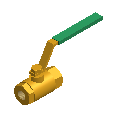
# Autodesk Inventor part: Parker Female-Female Pipe Ends XV500P XV500P-12
Saved by Autodesk Inventor 2020 (Build 240152000, 152)
## iProperties
_DisabledCommands: 0
Created: 2009-02-04
Part Number: Parker Female-Female Pipe Ends XV500P XV500P-12
Material: Brass, Soft Yellow
Description: Female-Female Pipe Ends
Document SubType Name: Modeling
Standard: Parker
Designer: Demir Ali
Manufacturer: Parker
Language: en-US
Size Designation: XV500P-12
Categories: <MemberInstance><Categories><Category DisplayName="Tube &amp; Pipe" InternalName="4347fa0f-2144-441d-94cd-e3e15c92b736" Mnemonic="TUBEANDPIPE"><CategoryParameter DisplayName="InLineGroups" InternalName="d60be647-bc43-4c18-a13f-9fe4115f8e64" Mnemonic="INLINEGROUPS"/><CategoryParameter DisplayName="Number of Connections" InternalName="04e9c83a-9e20-4a98-a7e1-e8abe87a2846" Mnemonic="NUM_CONNECTIONS"/><CategoryParameter DisplayName="Angles" InternalName="0e0e4fa4-3bd3-4656-a22e-4e07c8c476f8" Mnemonic="ANGLES"><CategoryParameter DisplayName="Angle" InternalName="9188ad83-1b16-48b4-8b0a-76ce729dafa7" Mnemonic="ANGLE"/></CategoryParameter><CategoryParameter DisplayName="NameOfComponent" InternalName="9c74ad13-48a1-45fe-b0f7-5447561f444a" Mnemonic="NAMEOFCOMPONENT"/><CategoryParameter DisplayName="SKey" InternalName="3da84699-049a-4bc2-a65a-6696b77c242f" Mnemonic="SKEY"/><CategoryParameter DisplayName="ITEM-CODE" InternalName="99cc3b15-24d9-4d38-aac7-792cfbc57acf" Mnemonic="ITEMCODE"/><CategoryParameter DisplayName="ISOGEN Description" InternalName="7aa3ba45-b821-4467-8584-f9e6f15f2a7d" Mnemonic="ISOGENDESC"/><Category DisplayName="Fittings" InternalName="ed6b26c4-72b8-4f31-9b63-f85ae8f932e4" Mnemonic="FITTINGS"><CategoryParameter DisplayName="Connections" InternalName="dbd721e8-e885-4eea-9011-b5acfd9f61de" Mnemonic="FIT_CONNECTIONS"><CategoryParameter DisplayName="NominalSize" InternalName="3f94edc7-e459-48db-8f02-8eebf8cffccd" Mnemonic="NS"/><CategoryParameter DisplayName="FlipDirection" InternalName="d55dedc0-f14a-4283-86b4-a4eeb253c8aa" Mnemonic="FLIPDIRECTION"/><CategoryParameter DisplayName="DisplayName" InternalName="50f521dd-e050-43f7-9895-6b30ea7ed42e" Mnemonic="DISPLAYNAME"/><CategoryParameter DisplayName="Female" InternalName="b366bcb5-a500-4bad-84bb-22f956216d69" Mnemonic="FEMALE"/><CategoryParameter DisplayName="EndTreatment" InternalName="d7f11516-3374-45ca-b1c7-4b2d63244ae2" Mnemonic="ENDTREATMENT"/><CategoryParameter DisplayName="Fixed" InternalName="9142902a-6a8a-446d-9eb8-4b7ce7d245ef" Mnemonic="FIXED"/><CategoryParameter DisplayName="MaxEngagement" InternalName="34fdf028-8797-436e-ba07-ca3dee15bd9b" Mnemonic="MAXENGAGEMENT"/><CategoryParameter DisplayName="MinEngagement [% of MaxEngagement]" InternalName="7ec1bde5-73f0-45b1-98d8-365a6c67f8ad" Mnemonic="MINENGAGEMENT"/><CategoryParameter DisplayName="ScheduleNumber" InternalName="d6161c62-eb59-4495-a086-874847c10866" Mnemonic="SN"/><CategoryParameter DisplayName="Max Mating Pipe Size" InternalName="e73ef66b-c04b-45ac-9b32-f712653e25ee" Mnemonic="MXMPS"/><CategoryParameter DisplayName="Min Mating Pipe Size" InternalName="11f51b32-3e37-4310-abf7-f1318a1fd129" Mnemonic="MNMPS"/><CategoryParameter DisplayName="Cut Mating Pipe" InternalName="53a63a6e-53d8-4ca9-8880-037731d1cceb" Mnemonic="CMP"/><CategoryParameter DisplayName="Gender Neutral" InternalName="628bd5f1-acad-44e2-9d91-af996ab74fc2" Mnemonic="NEUTRAL"/></CategoryParameter><CategoryParameter DisplayName="Connections" InternalName="dbd721e8-e885-4eea-9011-b5acfd9f61de" Mnemonic="FIT_CONNECTIONS"><CategoryParameter DisplayName="NominalSize" InternalName="3f94edc7-e459-48db-8f02-8eebf8cffccd" Mnemonic="NS"/><CategoryParameter DisplayName="FlipDirection" InternalName="d55dedc0-f14a-4283-86b4-a4eeb253c8aa" Mnemonic="FLIPDIRECTION"/><CategoryParameter DisplayName="DisplayName" InternalName="50f521dd-e050-43f7-9895-6b30ea7ed42e" Mnemonic="DISPLAYNAME"/><CategoryParameter DisplayName="Female" InternalName="b366bcb5-a500-4bad-84bb-22f956216d69" Mnemonic="FEMALE"/><CategoryParameter DisplayName="EndTreatment" InternalName="d7f11516-3374-45ca-b1c7-4b2d63244ae2" Mnemonic="ENDTREATMENT"/><CategoryParameter DisplayName="Fixed" InternalName="9142902a-6a8a-446d-9eb8-4b7ce7d245ef" Mnemonic="FIXED"/><CategoryParameter DisplayName="MaxEngagement" InternalName="34fdf028-8797-436e-ba07-ca3dee15bd9b" Mnemonic="MAXENGAGEMENT"/><CategoryParameter DisplayName="MinEngagement [% of MaxEngagement]" InternalName="7ec1bde5-73f0-45b1-98d8-365a6c67f8ad" Mnemonic="MINENGAGEMENT"/><CategoryParameter DisplayName="ScheduleNumber" InternalName="d6161c62-eb59-4495-a086-874847c10866" Mnemonic="SN"/><CategoryParameter DisplayName="Max Mating Pipe Size" InternalName="e73ef66b-c04b-45ac-9b32-f712653e25ee" Mnemonic="MXMPS"/><CategoryParameter DisplayName="Min Mating Pipe Size" InternalName="11f51b32-3e37-4310-abf7-f1318a1fd129" Mnemonic="MNMPS"/><CategoryParameter DisplayName="Cut Mating Pipe" InternalName="53a63a6e-53d8-4ca9-8880-037731d1cceb" Mnemonic="CMP"/><CategoryParameter DisplayName="Gender Neutral" InternalName="628bd5f1-acad-44e2-9d91-af996ab74fc2" Mnemonic="NEUTRAL"/></CategoryParameter><Category DisplayName="Valves" InternalName="b54f24b4-8c71-4f76-b075-760a31c67e8e" Mnemonic="Valve"/></Category></Category><Category DisplayName="DataType" InternalName="23b78d0f-2648-40c6-8793-ca6db495c9e8" Mnemonic="DATATYPE"><CategoryParameter DisplayName="DisplayName" InternalName="05415f3d-3907-474b-a020-eb9d644f4cf3" Mnemonic="DISPLAYNAME"/><CategoryParameter DisplayName="InternalName" InternalName="cf1d0246-76d9-4b4a-8305-fa0409afb5c1" Mnemonic="INTERNALNAME"/><CategoryParameter DisplayName="Folder Name" InternalName="3f06958e-8713-4116-9be7-ed6184ecc97b" Mnemonic="FOLDERNAME"/><CategoryParameter DisplayName="Family Version" InternalName="914462f6-6e19-4b14-ba84-155b9680b1d0" Mnemonic="FAMILYREVISION"/><CategoryParameter DisplayName="ClipFormat" InternalName="bc51e27b-3422-4e78-93ef-cec197ddf230" Mnemonic="CLIPFORMAT"/><CategoryParameter DisplayName="IsMetric" InternalName="e2385c5b-1ea4-4823-96a8-8de651266ec3" Mnemonic="ISMETRIC"/><CategoryParameter DisplayName="Description" InternalName="13903e3d-64b1-4950-80da-f627842ea37f" Mnemonic="DESCRIPTION"/><CategoryParameter DisplayName="StdsOrg" InternalName="8f5914e1-4693-403f-8ab5-d37768198c9d" Mnemonic="STDSORG"/><CategoryParameter DisplayName="Standard" InternalName="0c0a119c-1e12-4c84-803f-101930972f5e" Mnemonic="STANDARD"/><CategoryParameter DisplayName="Manufacturer" InternalName="cd6c7a72-a28a-4e50-99a9-2c7f4e13e5ad" Mnemonic="MANUFACTURER"/><CategoryParameter DisplayName="Member Revision" InternalName="a65d44b9-392f-4f4f-857b-e4b3d54996fe" Mnemonic="MEMBERREVISION"/><CategoryParameter DisplayName="Standard Revision" InternalName="91d5a463-65c2-4fde-b823-3b7fea5e8e17" Mnemonic="STANDARDREVISION"/><CategoryParameter DisplayName="Revision Guid" InternalName="45a75005-10b1-4dfc-8d6d-dfe629f0b93c" Mnemonic="REVISIONGUID"/><CategoryParameter DisplayName="Designation" InternalName="2675968c-4ce5-49e0-a4f5-552d29089031" Mnemonic="DESIGNATION"/><CategoryParameter DisplayName="FileName" InternalName="8b46a4cc-9585-4fed-90c3-899f57e09a73" Mnemonic="FILENAME"/><CategoryParameter DisplayName="Default Row" InternalName="2af9ec52-faaa-4026-b378-f9fa4afca842" Mnemonic="DEFAULTROW"/><Category DisplayName="Part" InternalName="c0e0b642-3bcb-4cc8-9e80-f96d35c4afa4" Mnemonic="PART"><CategoryParameter DisplayName="Material" InternalName="818a152a-d3c3-49ca-80ee-df7d91421b8e" Mnemonic="MATERIAL"/><CategoryParameter DisplayName="Material Key" InternalName="5c9a8adb-dd2b-4535-b97f-0a94a95fe41f" Mnemonic="MATERIALKEY"/><CategoryParameter DisplayName="Part Number" InternalName="016b6077-bfbe-49bd-92c9-d8d59c39c941" Mnemonic="PARTNUMBER"/><CategoryParameter DisplayName="Stock Number" InternalName="4dba7c1c-e26c-444e-836c-b08b433409a8" Mnemonic="STOCKNUMBER"/></Category></Category><Category DisplayName="LegacyMap" InternalName="dfeab48a-acc2-4514-a11c-1b8dc28c3d5f" Mnemonic="LEGACYMAP"><CategoryParameter DisplayName="CatalogID" InternalName="0da51c36-8fd3-4028-86cc-0c9c9e96136a" Mnemonic="CATALOGID"/><CategoryParameter DisplayName="FamilyID" InternalName="1c0b589c-8bbe-4e1e-80cf-07c0de42ac2a" Mnemonic="FAMILYID"/><CategoryParameter DisplayName="MemberID" InternalName="a368ea03-db8a-4d6e-962b-2aa46306b8f5" Mnemonic="MEMBERID"/></Category></Categories><FamilyTemplate Id="Parker Female-Female Pipe Ends XV500P"><FamilyTemplateParameters><FamilyTemplateParameter ObjectType="kUserParameterObject" ValueType="xs:double" Id="1" ObjectReferenceKey="D"/><FamilyTemplateParameter ObjectType="kUserParameterObject" ValueType="xs:double" Id="2" ObjectReferenceKey="N1"/><FamilyTemplateParameter ObjectType="kUserParameterObject" ValueType="xs:double" Id="3" ObjectReferenceKey="M"/><FamilyTemplateParameter ObjectType="kUserParameterObject" ValueType="xs:double" Id="4" ObjectReferenceKey="H1"/><FamilyTemplateParameter ObjectType="kUserParameterObject" ValueType="xs:double" Id="5" ObjectReferenceKey="L"/><FamilyTemplateParameter ObjectType="kUserParameterObject" ValueType="xs:double" Id="6" ObjectReferenceKey="B_HEX"/><FamilyTemplateParameter ObjectType="kUserParameterObject" ValueType="xs:double" Id="7" ObjectReferenceKey="C_HEX"/><FamilyTemplateParameter ObjectType="kUserParameterObject" ValueType="xs:string" Id="118" ObjectReferenceKey="Parker_No"/><FamilyTemplateParameter ObjectType="kPropertyObject" ValueType="xs:string" Id="100" ObjectReferenceKey="{32853F0F-3444-11d1-9E93-0060B03C1CA6}" SubObjectId="52"/><FamilyTemplateParameter ObjectType="kPropertyObject" ValueType="xs:string" Id="105" ObjectReferenceKey="{32853F0F-3444-11d1-9E93-0060B03C1CA6}" SubObjectId="5"/><FamilyTemplateParameter ObjectType="kPartComponentDefinitionObject" ValueType="xs:string" Id="110" SubObjectId="Material"/><FamilyTemplateParameter ObjectType="kThreadFeatureObject" ValueType="xs:structure" Id="300" ObjectReferenceKey="10020000100000002B880000000000008000000000000000" SubObjectId="ThreadInfo"><FamilyTemplateParameter ObjectType="" ValueType="xs:string" Id="301" SubObjectId="ThreadType"/><FamilyTemplateParameter ObjectType="" ValueType="xs:string" Id="302" SubObjectId="NominalDiameter"/></FamilyTemplateParameter><FamilyTemplateParameter ObjectType="kThreadFeatureObject" ValueType="xs:structure" Id="303" ObjectReferenceKey="100200001000000095880000000000008000000000000000" SubObjectId="ThreadInfo"><FamilyTemplateParameter ObjectType="" ValueType="xs:string" Id="304" SubObjectId="ThreadType"/><FamilyTemplateParameter ObjectType="" ValueType="xs:string" Id="305" SubObjectId="NominalDiameter"/></FamilyTemplateParameter></FamilyTemplateParameters></FamilyTemplate><CategoryParameterMap><ParamToTemplateMap><ParamToTemplate CategoryParameter="//CategoryParameter[@InternalName='d60be647-bc43-4c18-a13f-9fe4115f8e64']" ConstantValue="1"/><ParamToTemplate CategoryParameter="//CategoryParameter[@InternalName='04e9c83a-9e20-4a98-a7e1-e8abe87a2846']" ConstantValue="2"/><ParamToTemplate CategoryParameter="//CategoryParameter[@InternalName='0e0e4fa4-3bd3-4656-a22e-4e07c8c476f8']" ConstantValue=""/><ParamToTemplate CategoryParameter="//CategoryParameter[@InternalName='0e0e4fa4-3bd3-4656-a22e-4e07c8c476f8'][1]/CategoryParameter[@InternalName='9188ad83-1b16-48b4-8b0a-76ce729dafa7']" ConstantValue="3.14159265358979"/><ParamToTemplate CategoryParameter="//CategoryParameter[@InternalName='9c74ad13-48a1-45fe-b0f7-5447561f444a']" ConstantValue="VALVE"/><ParamToTemplate CategoryParameter="//CategoryParameter[@InternalName='3da84699-049a-4bc2-a65a-6696b77c242f']" ConstantValue="VBSC"/><ParamToTemplate CategoryParameter="//CategoryParameter[@InternalName='dbd721e8-e885-4eea-9011-b5acfd9f61de'][1]/CategoryParameter[@InternalName='d55dedc0-f14a-4283-86b4-a4eeb253c8aa']" ConstantValue="false"/><ParamToTemplate CategoryParameter="//CategoryParameter[@InternalName='dbd721e8-e885-4eea-9011-b5acfd9f61de'][1]/CategoryParameter[@InternalName='50f521dd-e050-43f7-9895-6b30ea7ed42e']" ConstantValue="Connection1"/><ParamToTemplate CategoryParameter="//CategoryParameter[@InternalName='dbd721e8-e885-4eea-9011-b5acfd9f61de'][1]/CategoryParameter[@InternalName='b366bcb5-a500-4bad-84bb-22f956216d69']" ConstantValue="true"/><ParamToTemplate CategoryParameter="//CategoryParameter[@InternalName='dbd721e8-e885-4eea-9011-b5acfd9f61de'][1]/CategoryParameter[@InternalName='d7f11516-3374-45ca-b1c7-4b2d63244ae2']" ConstantValue="Threaded"/><ParamToTemplate CategoryParameter="//CategoryParameter[@InternalName='dbd721e8-e885-4eea-9011-b5acfd9f61de'][1]/CategoryParameter[@InternalName='9142902a-6a8a-446d-9eb8-4b7ce7d245ef']" ConstantValue="false"/><ParamToTemplate CategoryParameter="//CategoryParameter[@InternalName='dbd721e8-e885-4eea-9011-b5acfd9f61de'][1]/CategoryParameter[@InternalName='34fdf028-8797-436e-ba07-ca3dee15bd9b']" ConstantValue="0"/><ParamToTemplate CategoryParameter="//CategoryParameter[@InternalName='dbd721e8-e885-4eea-9011-b5acfd9f61de'][1]/CategoryParameter[@InternalName='7ec1bde5-73f0-45b1-98d8-365a6c67f8ad']" ConstantValue="50"/><ParamToTemplate CategoryParameter="//CategoryParameter[@InternalName='dbd721e8-e885-4eea-9011-b5acfd9f61de'][2]/CategoryParameter[@InternalName='d55dedc0-f14a-4283-86b4-a4eeb253c8aa']" ConstantValue="false"/><ParamToTemplate CategoryParameter="//CategoryParameter[@InternalName='dbd721e8-e885-4eea-9011-b5acfd9f61de'][2]/CategoryParameter[@InternalName='50f521dd-e050-43f7-9895-6b30ea7ed42e']" ConstantValue="Connection2"/><ParamToTemplate CategoryParameter="//CategoryParameter[@InternalName='dbd721e8-e885-4eea-9011-b5acfd9f61de'][2]/CategoryParameter[@InternalName='b366bcb5-a500-4bad-84bb-22f956216d69']" ConstantValue="true"/><ParamToTemplate CategoryParameter="//CategoryParameter[@InternalName='dbd721e8-e885-4eea-9011-b5acfd9f61de'][2]/CategoryParameter[@InternalName='d7f11516-3374-45ca-b1c7-4b2d63244ae2']" ConstantValue="Threaded"/><ParamToTemplate CategoryParameter="//CategoryParameter[@InternalName='dbd721e8-e885-4eea-9011-b5acfd9f61de'][2]/CategoryParameter[@InternalName='9142902a-6a8a-446d-9eb8-4b7ce7d245ef']" ConstantValue="false"/><ParamToTemplate CategoryParameter="//CategoryParameter[@InternalName='dbd721e8-e885-4eea-9011-b5acfd9f61de'][2]/CategoryParameter[@InternalName='34fdf028-8797-436e-ba07-ca3dee15bd9b']" ConstantValue="0"/><ParamToTemplate CategoryParameter="//CategoryParameter[@InternalName='dbd721e8-e885-4eea-9011-b5acfd9f61de'][2]/CategoryParameter[@InternalName='7ec1bde5-73f0-45b1-98d8-365a6c67f8ad']" ConstantValue="50"/><ParamToTemplate CategoryParameter="//CategoryParameter[@InternalName='05415f3d-3907-474b-a020-eb9d644f4cf3']" ConstantValue="Parker Female-Female Pipe Ends XV500P"/><ParamToTemplate CategoryParameter="//CategoryParameter[@InternalName='cf1d0246-76d9-4b4a-8305-fa0409afb5c1']" ConstantValue="c0da0a2f-7571-4003-bdb7-f2d41c6df3db"/><ParamToTemplate CategoryParameter="//CategoryParameter[@InternalName='3f06958e-8713-4116-9be7-ed6184ecc97b']" ConstantValue="Parker XV500P"/><ParamToTemplate CategoryParameter="//CategoryParameter[@InternalName='914462f6-6e19-4b14-ba84-155b9680b1d0']" ConstantValue="10"/><ParamToTemplate CategoryParameter="//CategoryParameter[@InternalName='13903e3d-64b1-4950-80da-f627842ea37f']" ConstantValue="Female-Female Pipe Ends"/><ParamToTemplate CategoryParameter="//CategoryParameter[@InternalName='8f5914e1-4693-403f-8ab5-d37768198c9d']" TemplateParameter="101"/><ParamToTemplate CategoryParameter="//CategoryParameter[@InternalName='0c0a119c-1e12-4c84-803f-101930972f5e']" ConstantValue="Parker"/><ParamToTemplate CategoryParameter="//CategoryParameter[@InternalName='cd6c7a72-a28a-4e50-99a9-2c7f4e13e5ad']" ConstantValue="Parker"/><ParamToTemplate CategoryParameter="//CategoryParameter[@InternalName='91d5a463-65c2-4fde-b823-3b7fea5e8e17']" TemplateParameter="103"/><ParamToTemplate CategoryParameter="//CategoryParameter[@InternalName='bc51e27b-3422-4e78-93ef-cec197ddf230']" ConstantValue="CF_INVENTOR.STDPARTS"/><ParamToTemplate CategoryParameter="//CategoryParameter[@InternalName='e2385c5b-1ea4-4823-96a8-8de651266ec3']" ConstantValue="false"/><ParamToTemplate CategoryParameter="//CategoryParameter[@InternalName='45a75005-10b1-4dfc-8d6d-dfe629f0b93c']" ConstantValue="d42680ee-8555-4a0a-a7e5-a56780419997"/><ParamToTemplate CategoryParameter="//CategoryParameter[@InternalName='2af9ec52-faaa-4026-b378-f9fa4afca842']" ConstantValue="1"/><ParamToTemplate CategoryParameter="//CategoryParameter[@InternalName='0da51c36-8fd3-4028-86cc-0c9c9e96136a']" ConstantValue="FD8AAA93-B897-476C-BD5D-67C712EC5ABF"/><ParamToTemplate CategoryParameter="//CategoryParameter[@InternalName='1c0b589c-8bbe-4e1e-80cf-07c0de42ac2a']" ConstantValue="c0da0a2f-7571-4003-bdb7-f2d41c6df3db"/><ParamToTemplate CategoryParameter="//CategoryParameter[@InternalName='99cc3b15-24d9-4d38-aac7-792cfbc57acf']" ConstantValue=""/><ParamToTemplate CategoryParameter="//CategoryParameter[@InternalName='7aa3ba45-b821-4467-8584-f9e6f15f2a7d']" ConstantValue=""/><ParamToTemplate CategoryParameter="//CategoryParameter[@InternalName='dbd721e8-e885-4eea-9011-b5acfd9f61de'][1]/CategoryParameter[@InternalName='3f94edc7-e459-48db-8f02-8eebf8cffccd']" ConstantValue="3/4"/><ParamToTemplate CategoryParameter="//CategoryParameter[@InternalName='dbd721e8-e885-4eea-9011-b5acfd9f61de'][2]/CategoryParameter[@InternalName='3f94edc7-e459-48db-8f02-8eebf8cffccd']" ConstantValue="3/4"/><ParamToTemplate CategoryParameter="//CategoryParameter[@InternalName='8b46a4cc-9585-4fed-90c3-899f57e09a73']" ConstantValue="Parker Female-Female Pipe Ends XV500P XV500P-12"/><ParamToTemplate CategoryParameter="//CategoryParameter[@InternalName='a65d44b9-392f-4f4f-857b-e4b3d54996fe']" ConstantValue="c6e430e8-bfa0-4268-b118-467858021bfb"/><ParamToTemplate CategoryParameter="//CategoryParameter[@InternalName='a368ea03-db8a-4d6e-962b-2aa46306b8f5']" ConstantValue="45871262-182C-4A3A-B761-B256B8A1EA76"/><ParamToTemplate CategoryParameter="//CategoryParameter[@InternalName='2675968c-4ce5-49e0-a4f5-552d29089031']" TemplateParameter="100"/><ParamToTemplate CategoryParameter="//CategoryParameter[@InternalName='818a152a-d3c3-49ca-80ee-df7d91421b8e']" TemplateParameter="110"/><ParamToTemplate CategoryParameter="//CategoryParameter[@InternalName='016b6077-bfbe-49bd-92c9-d8d59c39c941']" TemplateParameter="105"/></ParamToTemplateMap></CategoryParameterMap></MemberInstance>
Density: 8.47 g/cm^3
Mass: 491.245 g
Surface Area: 182.511 cm^2
Volume: 57.9983 cm^3
Appearance: Brass - Satin
NAME: PIPING: Parker Female-Female Pipe Ends XV500P
DATA: <meta><inlinegroups number="1" deflen="5.41401"></inlinegroups><connections number="2"></connections><angles><a>3.14159265358979</a></angles></meta>
IsCustomPart: 0
Author: Demir Ali
Autodesk Inventor part; units mm, degrees
sketch "Sketch3" plane through (0, 0, 0) normal (0, 1, 0) x (-1, 0, 0)
  circle A0 centre (0, 0) radius 10.7569
  dimension "d16" = 21.5138
  constraints: 1 centre point, 1 coincident
  measures "d16" diameter of A0
extrude "Extrusion3" add sketch "Sketch3" along normal blind 26.67
sketch "Sketch4" plane through (0, 26.67, 0) normal (0, 1, 0) x (1, 0, 0)
  circle A0 centre (0, 0) radius 10.7569 projected
  circle A1 centre (0, 0) radius 4.6101
  dimension "d19" = 9.2202
  constraints: 1 centre point, 1 coincident
  measures "d19" diameter of A1
extrude "Extrusion4" add sketch "Sketch4" along normal blind 0.7137 contours A1
sketch "Sketch5" plane through (0, 27.3837, 0) normal (0, 1, 0) x (1, 0, 0)
  circle A0 centre (0, 0) radius 4.6101 projected
  circle A1 centre (0, 0) radius 6.1468
  dimension "d22" = 12.2936
  constraints: 1 centre point, 1 coincident
  measures "d22" diameter of A1
extrude "Extrusion5" add sketch "Sketch5" along normal blind 1.4275 contours A0 | A1
sketch "Sketch6" plane through (0, 28.8112, 0) normal (0, 1, 0) x (1, 0, 0)
  circle A0 centre (0, 0) radius 6.1468 projected
  circle A1 centre (0, 0) radius 2.4587
  dimension "d25" = 4.9174
  constraints: 1 centre point, 1 coincident
  measures "d25" diameter of A1
extrude "Extrusion6" add sketch "Sketch6" along normal mid plane 14.2748 contours A1
sketch "Sketch7" plane through (0, 35.9486, 0) normal (0, 1, 0) x (1, 0, 0)
  circle A0 centre (0, 0) radius 2.4587 projected
  line L0 (9.1654, 0) -> (4.5827, -7.9375)
  line L1 (4.5827, -7.9375) -> (-4.5827, -7.9375)
  line L2 (-4.5827, -7.9375) -> (-9.1654, 0)
  line L3 (-9.1654, 0) -> (-4.5827, 7.9375)
  line L4 (-4.5827, 7.9375) -> (4.5827, 7.9375)
  line L5 (4.5827, 7.9375) -> (9.1654, 0)
  dimension "d28" = 15.875
  constraints: 12 end point, 1 coincident, 11 other
  measures "d28" distance between parallel lines of L1 L4
extrude "Extrusion7" add sketch "Sketch7" against normal blind 4.9962 contours A0 | L0 L1 L2 L3 L4 L5
sketch "Sketch8" plane through (0, 0, 0) normal (1, 0, 0) x (0, 1, 0)
  line L0 (30.9524, 7.9375) -> (30.9524, 0) projected
  line L1 (30.9524, 8.6055) -> (30.9524, -7.9908)
  line L2 (30.9524, -7.9908) -> (54.6665, -21.6822)
  line L3 (54.6665, -21.6822) -> (54.6665, -100.584)
  line L4 (51.0978, -100.584) -> (51.0978, -23.7426)
  line L5 (51.0978, -23.7426) -> (27.3837, -10.0512)
  line L6 (27.3837, -10.0512) -> (27.3837, 8.6055)
  line L7 (54.6665, -100.584) -> (51.0978, -100.584)
  line L8 (30.9524, 8.6055) -> (27.3837, 8.6055)
  line L9 (35.9486, 0) -> (30.9524, 0) projected
  line L10 (0, 10.7569) -> (0, -10.7569) projected
  dimension "d31" = 3.5687
  dimension "d32" = 8.6055
  dimension "d33" = 120
  dimension "d34" = 100.584
  dimension "d36" = 7.9908
  dimension "d54" = 54.6665
  constraints: 16 end point, 2 parallel, 1 collinear, 1 perpendicular, 1 point on line, 2 other
  measures "d31" distance between parallel lines of L3 L4
  measures "d32" distance between parallel lines of L8 L9
  measures "d33" angle of L2 L1
  measures "d34" distance between parallel lines of L7 L9
  measures "d36" distance from line of L1.end L9
  measures "d54" distance between parallel lines of L3 L10
extrude "Extrusion8" add sketch "Sketch8" along normal mid plane 10.0584
sketch "Sketch9" plane through (0, 26.67, 0) normal (0, 1, 0) x (1, 0, 0)
  circle A0 centre (0, 0) radius 10.7569 projected
  line L0 (0, -10.7569) -> (0, 1.5367)
  line L1 (0, 1.5367) -> (-10.6466, 1.5367)
  circle A1 centre (0, 0) radius 4.6101 projected
  dimension "d73" = 12.2936
  constraints: 4 end point, 2 point on circle, 2 point on line, 1 perpendicular, 1 vertical
  measures "d73" distance of L0.start L0.end
extrude "Extrusion9" cut sketch "Sketch9" against normal blind 5.7099 contours L1 A1 L0 A0 | L1 L0 A1 picked at (-1.2328, -8.5574) picked at (-0.3635, -2.5175)
ref_plane "Work Plane2" through (0, 0, -24.5872) normal (0, 0, 1) x (1, 0, 0)
sketch "Sketch15" plane through (-5.0292, 27.3837, 8.6055) normal (0, -1, 0) x (1, 0, 0)
  line L0 (10.0584, 0) -> (0, 0) projected
  line L1 (5.0292, 0) -> (3.4925, 0)
  line L2 (3.4925, 0) -> (3.4925, -2.1514)
  line L3 (3.4925, -2.1514) -> (5.0292, -2.1514)
  line L4 (5.0292, 0) -> (5.0292, -2.1514)
  line L5 (5.0292, -131.4577) -> (5.0292, 24.4196) projected
  dimension "d63" = 2.1514
  dimension "d74" = 1.5367
  constraints: 8 end point, 2 perpendicular, 1 collinear, 1 midpoint, 1 point on line
  measures "d63" distance of L1.end L2.end
  measures "d74" distance between parallel lines of L4 L2
extrude "Extrusion15" add sketch "Sketch15" along normal blind 5.7099
sketch "Sketch16" plane through (0, 0, 0) normal (0, 1, 0) x (-1, 0, 0)
  circle A0 centre (0, 0) radius 2.0625 projected
extrude "Extrusion16" add sketch "Sketch16" along normal blind 28.5496
sketch "Sketch20" plane through (0, 0, 0) normal (1, 0, 0) x (0, 1, 0)
  line L0 (35.9486, 7.9375) -> (30.9524, 7.9375) projected
  line L1 (35.9486, 7.9375) -> (35.9486, 9.365)
  line L2 (35.9486, 9.365) -> (35.283, 9.365)
  line L3 (35.283, 9.365) -> (35.9486, 7.9375)
  line L4 (-7.1897, 0) -> (43.1383, 0) projected
  dimension "d94" = 1.4275
  dimension "d95" = 25
  constraints: 6 end point, 2 perpendicular
  measures "d94" distance of L0.start L1.end
  measures "d95" angle of L1 L3
ref_plane "Work Plane5" through (4.5827, 33.4505, 7.9375) normal (0, 1, 0) x (0.5, 0, -0.866)
revolve "Revolution3" cut sketch "Sketch20" angle 360 about axis through (0, -10, 0) along (0, 1, 0)
ref_plane "Work Plane6" through (0, 0, 32.766) normal (0, 0, 1) x (1, 0, 0)
ref_plane "Work Plane9" through (0, 0, 32.766) normal (0, 0, 1) x (1, 0, 0)
sketch "Sketch29" plane through (0, 0, 32.766) normal (0, 0, 1) x (1, 0, 0)
  line L0 (0, 19.2474) -> (16.6688, 9.6237)
  line L1 (16.6688, 9.6237) -> (16.6688, -9.6237)
  line L2 (16.6688, -9.6237) -> (0, -19.2474)
  line L3 (0, -19.2474) -> (-16.6687, -9.6237)
  line L4 (-16.6687, -9.6237) -> (-16.6688, 9.6237)
  line L5 (-16.6688, 9.6237) -> (0, 19.2474)
  point P0 (0, 0)
  point P1 (0, 0)
  point P2 (16.6687, 0)
  dimension "d140" = 33.3375
  constraints: 12 end point, 1 coincident, 1 horizontal alignment, 1 midpoint, 11 other
  measures "d140" distance between parallel lines of L4 L1
extrude "Extrusion23" add sketch "Sketch29" against normal blind 9.2202
sketch "Sketch30" plane through (0, 0, 23.5458) normal (0, 0, -1) x (-1, 0, 0)
  line L0 (16.6688, 9.6237) -> (16.6687, -9.6237) projected
  line L1 (0, 19.2474) -> (0, -19.2474)
  circle A0 centre (0, 0) radius 19.2474
  constraints: 2 end point, 1 midpoint, 1 parallel, 1 vertical alignment, 2 other
extrude "Extrusion24" add sketch "Sketch30" along normal blind 39.9542
sketch "Sketch31" plane through (0, 0, -16.4084) normal (0, 0, -1) x (-1, 0, 0)
  circle A0 centre (0, 0) radius 19.2474 projected
  line L0 (0, 18.3309) -> (15.875, 9.1654)
  line L1 (15.875, 9.1654) -> (15.875, -9.1654)
  line L2 (15.875, -9.1654) -> (0, -18.3309)
  line L3 (0, -18.3309) -> (-15.875, -9.1654)
  line L4 (-15.875, -9.1654) -> (-15.875, 9.1654)
  line L5 (-15.875, 9.1654) -> (0, 18.3309)
  point P0 (-15.875, 0)
  dimension "d145" = 31.75
  constraints: 12 end point, 1 coincident, 1 horizontal alignment, 1 midpoint, 11 other
  measures "d145" distance between parallel lines of L1 L4
extrude "Extrusion25" add sketch "Sketch31" along normal blind 15.367 contours L0 L1 L2 L3 L4 L5
hole "Hole4" at (0, 0, 32.766) direction (0, 0, -1) diameter 21.7488 depth 18.4404
hole "Hole5" at (0, 0, -31.7754) direction (0, 0, 1) diameter 21.7488 depth 18.4404
hole "Hole6" at (0, 0, 14.3256) direction (0, 0, -1) diameter 17.399 end through all
sketch "Sketch32" plane through (0, 0, 0) normal (0, 1, 0) x (-1, 0, 0)
  line L0 (16.6688, 32.766) -> (0, 32.766) projected
  line L1 (16.6688, 32.766) -> (24.6063, 32.766)
  line L2 (24.6063, 32.766) -> (24.6063, 29.0647)
  line L3 (24.6063, 29.0647) -> (16.6688, 32.766)
  line L4 (0, -6.5532) -> (0, 39.3192) projected
  dimension "d157" = 25
  dimension "d158" = 7.9375
  constraints: 6 end point, 1 collinear, 1 perpendicular
  measures "d157" angle of L1 L3
  measures "d158" distance of L0.start L1.end
revolve "Revolution6" cut sketch "Sketch32" angle 360 about axis through (0, 0, -10) along (0, 0, 1)
sketch "Sketch33" plane through (0, 0, 0) normal (0, 1, 0) x (-1, 0, 0)
  line L0 (0, -31.7754) -> (15.875, -31.7754) projected
  line L1 (15.875, -31.7754) -> (0, -31.7754) projected
  line L2 (0, -16.4084) -> (0, -31.7754) projected
  line L3 (15.875, -16.4084) -> (15.875, -31.7754) projected
  line L4 (15.875, -31.7754) -> (23.8125, -31.7754)
  line L5 (23.8125, -31.7754) -> (23.8125, -28.0741)
  line L6 (23.8125, -28.0741) -> (15.875, -31.7754)
  line L7 (0, -38.1305) -> (0, 6.3551) projected
  line L8 (15.875, -16.4084) -> (0, -16.4084) projected
  point P0 (0, -17.3736)
  dimension "d160" = 25
  dimension "d161" = 7.9375
  constraints: 6 end point, 2 perpendicular
  measures "d160" angle of L6 L4
  measures "d161" distance of L1.start L4.end
revolve "Revolution7" cut sketch "Sketch33" angle 360 about axis through (0, 0, -10) along (0, 0, 1) contours L6 L5 L4
sketch "Sketch34" plane through (5.0292, 51.0978, -100.584) normal (0, 0, -1) x (-1, 0, 0)
  line L0 (0, 3.5687) -> (0, 0) projected
  line L1 (0, 3.5687) -> (10.0584, 3.5687) projected
  line L2 (-0.7544, 4.4012) -> (10.8128, 4.4012)
  line L3 (10.8128, 4.4012) -> (10.8128, -0.628)
  line L4 (10.8128, -0.628) -> (-0.7544, -0.628)
  line L5 (-0.7544, -0.628) -> (-0.7544, 4.4012)
  point P0 (0, 1.7843)
  point P1 (-0.7544, 1.8866)
  point P2 (5.0292, 3.5687)
  point P3 (5.0292, 4.4012)
  point P4 (5.0292, -51.0978)
  dimension "d163" = 11.5672
  dimension "d164" = 5.0292
  dimension "d165" = 55.499
  constraints: 8 end point, 4 midpoint, 2 parallel, 1 horizontal, 1 perpendicular, 1 vertical alignment
  measures "d163" distance of L3.end L4.end
  measures "d164" distance of L4.end L2.start
  measures "d165" distance from line of L2 point (5.029, -51.098)
extrude "Extrusion26" add sketch "Sketch34" against normal blind 70.4088
thread "Thread4" size "3/4" designation "3/4 - 14 NPT" standard "NPT for PVC Pipe and Fitting" length 12.2936
thread "Thread5" size "3/4" designation "3/4 - 14 NPT" standard "NPT for PVC Pipe and Fitting" length 12.2936
equation "\"d16\" = 0.35 * M"
equation "\"d17\" = 0.8 * C_HEX"
equation "\"d19\" = 0.15 * M"
equation "\"d20\" = 0.01 * N1"
equation "\"d22\" = 0.2 * M"
equation "\"d23\" = 0.02 * N1"
equation "\"d25\" = 0.08 * M"
equation "\"d26\" = 0.2 * N1"
equation "\"d28\" = 0.5 * B_HEX"
equation "\"d29\" = 0.07 * N1"
equation "\"d31\" = 0.05 * N1"
equation "\"d32\" = 0.14 * M"
equation "\"d34\" = H1"
equation "\"d36\" = 0.13 * M"
equation "\"d54\" = -0.4925 * B_HEX + 0.985 * N1"
equation "\"d37\" = 0.1 * H1"
equation "\"d73\" = 0.2 * M"
equation "\"d39\" = 0.08 * N1"
equation "\"d63\" = 0.035 * M"
equation "\"d74\" = 0.025 * M"
equation "\"d64\" = 0.08 * N1"
equation "\"d75\" = 0.4 * N1"
equation "\"d94\" = 0.02 * N1"
equation "\"d140\" = C_HEX"
equation "\"d141\" = 0.15 * M"
equation "\"d143\" = 0.65 * M"
equation "\"d145\" = B_HEX"
equation "\"d146\" = 0.25 * M"
equation "\"d150\" = 1.25 * D"
equation "\"d155\" = 0.3 * M"
equation "\"d178\" = d150"
equation "\"d183\" = 0.3 * M"
equation "\"d187\" = D"
equation "\"d192\" = 0.3 * M"
equation "\"d158\" = 0.25 * B_HEX"
equation "\"d161\" = 0.25 * B_HEX"
equation "\"d163\" = 0.115 * H1"
equation "\"d164\" = 0.05 * H1"
equation "\"d165\" = N1 - 0.5 * B_HEX"
equation "\"d166\" = 0.7 * H1"
equation "\"d170\" = 0.2 * M"
equation "\"d172\" = 0.2 * M"
equation "\"D\" = 17.399"
equation "\"N1\" = 71.374"
equation "\"M\" = 61.468"
equation "\"H1\" = 100.584"
equation "\"L\" = 133.35"
equation "\"B_HEX\" = 31.75"
equation "\"C_HEX\" = 33.3375"
equation "\"d41\" = -0.4 * M"
equation "\"d104\" = L - H1"
equation "\"d139\" = L - H1"
equation "\"P_TH\" = 6.35"
equation "\"Parker_No\" = 1.2345"
body "Solid1"
